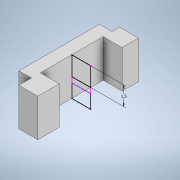
# Autodesk Inventor part: Button
Saved by Autodesk Inventor 2020 (Build 240168000, 168)
## iProperties
Created: 2021-08-24
Part Number: Button
Material: Generic
Document SubType Name: Modeling
Designer: nigel
Density: 1 g/cm^3
Appearance: Default
Author: nigel
Autodesk Inventor part; units mm, degrees
ref_plane "YZ Plane" through (0, 0, 0) normal (1, 0, 0) x (0, 1, 0)
ref_plane "XZ Plane" through (0, 0, 0) normal (0, 1, 0) x (-1, 0, 0)
ref_plane "XY Plane" through (0, 0, 0) normal (0, 0, 1) x (1, 0, 0)
sketch "Sketch1" plane through (0, 0, 0) normal (0, 1, 0) x (-1, 0, 0)
  line L0 (0.5, 3.2) -> (-0.5, 3.2)
  line L1 (-0.5, 3.2) -> (-0.5, -3.2)
  line L2 (-0.5, -3.2) -> (0.5, -3.2)
  line L3 (0.5, -3.2) -> (0.5, 3.2)
  line L4 (0.5, 3.2) -> (-0.5, -3.2) construction
  line L5 (-0.5, 3.2) -> (0.5, -3.2) construction
  line L6 (-0.5, -1.3) -> (-2, -1.3) construction
  line L7 (-2, -1.3) -> (-2, -3.4525)
  line L8 (-0.5, -3.2) -> (-0.5, -1.3)
  line L9 (-2, -3.4525) -> (-2, -3.8)
  line L10 (-2, -3.8) -> (-0.5, -3.8)
  line L11 (-0.5, -3.8) -> (-0.5, -3.2)
  line L12 (-2, -2.5) -> (-0.5, -2.5)
  line L13 (0, 0) -> (-4.1965, 0) construction
  line L14 (-2, 1.3) -> (-2, 3.4525)
  line L15 (-2, 2.5) -> (-0.5, 2.5)
  line L16 (-0.5, 2.5) -> (-2, 2.5)
  line L17 (-2, 2.5) -> (-2, 4.2)
  line L18 (-2, 4.2) -> (-0.5, 4.2)
  line L19 (-0.5, 4.2) -> (-0.5, 2.5)
  point P0 (-0.5, 3.2)
  dimension "d0" = 1.3
  dimension "d2" = 1
  dimension "d3" = 1.5
  dimension "d5" = 1.9
  dimension "d7" = 2.5
  dimension "d13" = 1
  dimension "d14" = 2.5
  constraints: 40 end point, 6 parallel, 5 point on line, 4 horizontal, 4 perpendicular, 4 symmetric about line, 2 midpoint, 1 collinear, 1 vertical
  measures "d0" distance from line of L13.start L6
  measures "d2" distance between parallel lines of L3 L1
  measures "d3" distance between parallel lines of L1 L7
  measures "d5" distance between parallel lines of L2 L6
  measures "d7" distance from line of L13.start L12
  measures "d13" distance between parallel lines of L0 L18
  measures "d14" distance between parallel lines of L6 L10
extrude "Extrusion1" add sketch "Sketch1" along normal blind 3
sketch "Sketch2" plane through (0, 0, 0) normal (0, 0, 1) x (1, 0, 0)
  line L0 (0.5, 0) -> (0.5, 3) projected
  line L1 (0.5, 3) -> (2, 3)
  line L2 (2, 3) -> (2, 1.5)
  line L3 (2, 1.5) -> (0.5, 1.5)
  line L4 (0.5, 1.5) -> (0.5, 3)
  line L5 (0.5, 0) -> (2, 0)
  line L6 (2, 0) -> (2, 1.0772)
  line L7 (2, 1.0772) -> (0.5, 1.0772)
  line L8 (0.5, 1.0772) -> (0.5, 0)
  line L9 (2, 0) -> (2, 3) projected
  point P0 (0, 0)
  dimension "d11" = 1.5
  constraints: 16 end point, 4 parallel, 2 horizontal, 2 perpendicular, 1 midpoint, 1 point on line
  measures "d11" distance between parallel lines of L1 L3
equation "\"button_height\" = 1.3"
body "Solid1"
